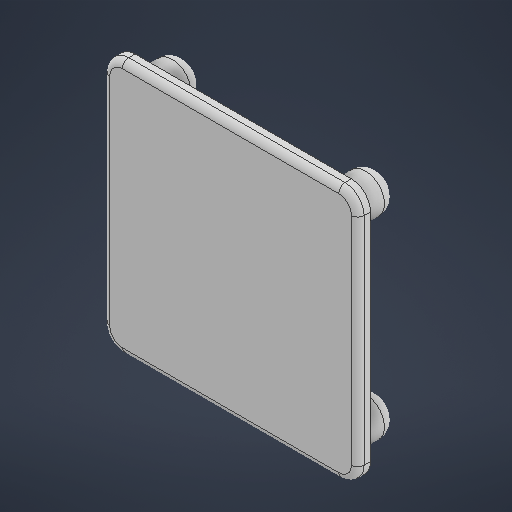
# Autodesk Inventor part: затычка
Saved by Autodesk Inventor 2025 (Build 290162000, 162)
## iProperties
Created: 2024-12-14
Part Number: затычка
Material: Типовые
Document SubType Name: Modeling
Designer: Phantom
Density: 1 g/cm^3
Appearance: По умолчанию
Author: Phantom
Autodesk Inventor part; units mm, degrees
ref_plane "YZ Plane" through (0, 0, 0) normal (1, 0, 0) x (0, 1, 0)
ref_plane "XZ Plane" through (0, 0, 0) normal (0, 1, 0) x (-1, 0, 0)
ref_plane "XY Plane" through (0, 0, 0) normal (0, 0, 1) x (1, 0, 0)
sketch "Эскиз1" plane through (0, 0, 0) normal (0, 0, 1) x (1, 0, 0)
  circle A0 centre (0, 0) radius 2.5
  circle A1 centre (7.6, 7.6) radius 1.5
  circle A2 centre (-7.6, 7.6) radius 1.5
  circle A3 centre (-7.6, -7.6) radius 1.5
  circle A4 centre (7.6, -7.6) radius 1.5
  arc A5 (-8.5, 10) -> (-10, 8.5) centre (-8.5, 8.5) ccw
  line L0 (-8.5, 10) -> (8.5, 10)
  line L1 (-10, -8.5) -> (-10, 8.5)
  line L2 (-10, -8.5) -> (-10, -3.95)
  arc A6 (-10, -8.5) -> (-8.5, -10) centre (-8.5, -8.5) ccw
  line L3 (-3.95, -10) -> (-8.5, -10)
  line L4 (8.5, -10) -> (-8.5, -10)
  arc A7 (8.5, -10) -> (10, -8.5) centre (8.5, -8.5) ccw
  line L5 (10, -3.95) -> (10, -8.5)
  line L6 (10, 8.5) -> (10, -8.5)
  arc A8 (10, 8.5) -> (8.5, 10) centre (8.5, 8.5) ccw
  line L7 (3.95, 10) -> (8.5, 10)
  constraints: 16 end point, 9 centre point, 8 point on circle, 1 coincident
extrude "Выдавливание1" add sketch "Эскиз1" along normal blind 1 contours A0 | A1 | A2 | A3 | A4 | L0 A8 L6 L5 A7 L4 L3 A6 L1 A5
fillet "Сопряжение1" radius 0.5 11 edges at (-9.5607, -9.5607, 1) (0, -10, 1) (9.5607, -9.5607, 1) (10, 2.275, 1) (10, -6.225, 1) (9.5607, 9.5607, 1) (-2.275, 10, 1) (6.225, 10, 1) (-9.5607, 9.5607, 1) (-10, -6.225, 1) (-10, 2.275, 1)
sketch "Эскиз2" plane through (0, 0, 0) normal (0, 0, -1) x (-1, 0, 0)
  circle A0 centre (0, 0) radius 2.5
  circle A1 centre (7.6, 7.6) radius 1.5
  circle A2 centre (-7.6, 7.6) radius 1.5
  circle A3 centre (-7.6, -7.6) radius 1.5
  circle A4 centre (7.6, -7.6) radius 1.5
  constraints: 5 centre point, 1 coincident
extrude "Выдавливание2" add sketch "Эскиз2" along normal blind 3
fillet "Сопряжение2" radius 1 5 edges at (-6.1, -7.6, -3) (9.1, -7.6, -3) (2.5, 0, -3) (-6.1, 7.6, -3) (9.1, 7.6, -3)
